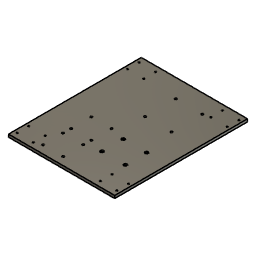
Base roulante (Autodesk Fusion 360 design; units mm, degrees)
Autodesk Fusion 360 part; units mm, degrees
sketch "Sketch1" plane through (0, 0, 0) normal (0, 1, 0) x (1, 0, 0)
  line L0 (0, 0) -> (200, 0)
  line L1 (200, 0) -> (200, 250)
  line L2 (200, 250) -> (0, 250)
  line L3 (0, 250) -> (0, 0)
  circle A0 centre (6, 240) radius 1.5
  circle A1 centre (37, 240) radius 1.5
  line L4 (100, 250) -> (100, 0)
  line L5 (0, 125) -> (200, 125)
  circle A2 centre (163, 240) radius 1.5
  circle A3 centre (194, 240) radius 1.5
  circle A4 centre (6, 10) radius 1.5
  circle A5 centre (163, 10) radius 1.5
  circle A6 centre (37, 10) radius 1.5
  circle A7 centre (194, 10) radius 1.5
  circle A8 centre (6, 218) radius 1.5
  circle A9 centre (37, 218) radius 1.5
  circle A10 centre (163, 218) radius 1.5
  circle A11 centre (194, 218) radius 1.5
  circle A12 centre (37, 32) radius 1.5
  circle A13 centre (6, 32) radius 1.5
  circle A14 centre (194, 32) radius 1.5
  circle A15 centre (163, 32) radius 1.5
  line L6 (34.25, 238.4123) -> (37, 236.8246)
  line L7 (37, 236.8246) -> (39.75, 238.4123)
  line L8 (39.75, 238.4123) -> (39.75, 241.5877)
  line L9 (39.75, 241.5877) -> (37, 243.1754)
  line L10 (37, 243.1754) -> (34.25, 241.5877)
  line L11 (34.25, 241.5877) -> (34.25, 238.4123)
  line L12 (8.75, 238.4123) -> (8.75, 241.5877)
  line L13 (8.75, 241.5877) -> (6, 243.1754)
  line L14 (6, 243.1754) -> (3.25, 241.5877)
  line L15 (3.25, 241.5877) -> (3.25, 238.4123)
  line L16 (3.25, 238.4123) -> (6, 236.8246)
  line L17 (6, 236.8246) -> (8.75, 238.4123)
  line L18 (34.25, 219.5877) -> (34.25, 216.4123)
  line L19 (34.25, 216.4123) -> (37, 214.8246)
  line L20 (37, 214.8246) -> (39.75, 216.4123)
  line L21 (39.75, 216.4123) -> (39.75, 219.5877)
  line L22 (39.75, 219.5877) -> (37, 221.1754)
  line L23 (37, 221.1754) -> (34.25, 219.5877)
  line L24 (3.25, 219.5877) -> (3.25, 216.4123)
  line L25 (3.25, 216.4123) -> (6, 214.8246)
  line L26 (6, 214.8246) -> (8.75, 216.4123)
  line L27 (8.75, 216.4123) -> (8.75, 219.5877)
  line L28 (8.75, 219.5877) -> (6, 221.1754)
  line L29 (6, 221.1754) -> (3.25, 219.5877)
  line L30 (191.25, 238.4123) -> (191.25, 241.5877)
  line L31 (194, 214.8246) -> (191.25, 216.4123)
  line L32 (160.25, 219.5877) -> (163, 221.1754)
  line L33 (163, 214.8246) -> (160.25, 216.4123)
  line L34 (163, 236.8246) -> (160.25, 238.4123)
  line L35 (194, 221.1754) -> (196.75, 219.5877)
  line L36 (191.25, 219.5877) -> (194, 221.1754)
  line L37 (196.75, 219.5877) -> (196.75, 216.4123)
  line L38 (194, 236.8246) -> (191.25, 238.4123)
  line L39 (160.25, 238.4123) -> (160.25, 241.5877)
  line L40 (160.25, 216.4123) -> (160.25, 219.5877)
  line L41 (196.75, 238.4123) -> (194, 236.8246)
  line L42 (196.75, 216.4123) -> (194, 214.8246)
  line L43 (160.25, 241.5877) -> (163, 243.1754)
  line L44 (165.75, 219.5877) -> (165.75, 216.4123)
  line L45 (196.75, 241.5877) -> (196.75, 238.4123)
  line L46 (163, 221.1754) -> (165.75, 219.5877)
  line L47 (165.75, 216.4123) -> (163, 214.8246)
  line L48 (194, 243.1754) -> (196.75, 241.5877)
  line L49 (191.25, 216.4123) -> (191.25, 219.5877)
  line L50 (165.75, 238.4123) -> (163, 236.8246)
  line L51 (191.25, 241.5877) -> (194, 243.1754)
  line L52 (163, 243.1754) -> (165.75, 241.5877)
  line L53 (165.75, 241.5877) -> (165.75, 238.4123)
  line L54 (8.75, 33.5877) -> (8.75, 30.4123)
  line L55 (37, 28.8246) -> (34.25, 30.4123)
  line L56 (34.25, 8.4123) -> (34.25, 11.5877)
  line L57 (37, 35.1754) -> (39.75, 33.5877)
  line L58 (6, 35.1754) -> (8.75, 33.5877)
  line L59 (34.25, 33.5877) -> (37, 35.1754)
  line L60 (37, 6.8246) -> (34.25, 8.4123)
  line L61 (3.25, 8.4123) -> (3.25, 11.5877)
  line L62 (39.75, 11.5877) -> (39.75, 8.4123)
  line L63 (6, 13.1754) -> (8.75, 11.5877)
  line L64 (37, 13.1754) -> (39.75, 11.5877)
  line L65 (39.75, 8.4123) -> (37, 6.8246)
  line L66 (39.75, 30.4123) -> (37, 28.8246)
  line L67 (8.75, 11.5877) -> (8.75, 8.4123)
  line L68 (8.75, 30.4123) -> (6, 28.8246)
  line L69 (34.25, 11.5877) -> (37, 13.1754)
  line L70 (3.25, 30.4123) -> (3.25, 33.5877)
  line L71 (34.25, 30.4123) -> (34.25, 33.5877)
  line L72 (8.75, 8.4123) -> (6, 6.8246)
  line L73 (3.25, 33.5877) -> (6, 35.1754)
  line L74 (6, 6.8246) -> (3.25, 8.4123)
  line L75 (39.75, 33.5877) -> (39.75, 30.4123)
  line L76 (6, 28.8246) -> (3.25, 30.4123)
  line L77 (3.25, 11.5877) -> (6, 13.1754)
  line L78 (191.25, 8.4123) -> (194, 6.8246)
  line L79 (165.75, 11.5877) -> (163, 13.1754)
  line L80 (194, 6.8246) -> (196.75, 8.4123)
  line L81 (165.75, 30.4123) -> (165.75, 33.5877)
  line L82 (163, 28.8246) -> (165.75, 30.4123)
  line L83 (196.75, 11.5877) -> (194, 13.1754)
  line L84 (191.25, 30.4123) -> (194, 28.8246)
  line L85 (194, 13.1754) -> (191.25, 11.5877)
  line L86 (196.75, 33.5877) -> (194, 35.1754)
  line L87 (165.75, 33.5877) -> (163, 35.1754)
  line L88 (194, 35.1754) -> (191.25, 33.5877)
  line L89 (165.75, 8.4123) -> (165.75, 11.5877)
  line L90 (160.25, 11.5877) -> (160.25, 8.4123)
  line L91 (196.75, 30.4123) -> (196.75, 33.5877)
  line L92 (163, 6.8246) -> (165.75, 8.4123)
  line L93 (160.25, 33.5877) -> (160.25, 30.4123)
  line L94 (163, 13.1754) -> (160.25, 11.5877)
  line L95 (191.25, 11.5877) -> (191.25, 8.4123)
  line L96 (196.75, 8.4123) -> (196.75, 11.5877)
  line L97 (160.25, 30.4123) -> (163, 28.8246)
  line L98 (160.25, 8.4123) -> (163, 6.8246)
  line L99 (191.25, 33.5877) -> (191.25, 30.4123)
  line L100 (163, 35.1754) -> (160.25, 33.5877)
  line L101 (194, 28.8246) -> (196.75, 30.4123)
  point P0 (37, 240)
  point P1 (6, 240)
  point P2 (37, 218)
  point P3 (6, 218)
  point P4 (194, 240)
  point P5 (163, 218)
  point P6 (163, 218)
  point P7 (194, 240)
  point P8 (194, 218)
  point P9 (6, 10)
  point P10 (37, 10)
  point P11 (37, 10)
  point P12 (6, 32)
  point P13 (6, 10)
  point P14 (6, 32)
  point P15 (37, 32)
  point P16 (37, 32)
  point P17 (194, 10)
  point P18 (163, 10)
  point P19 (194, 32)
  point P20 (163, 32)
  point P21 (163, 32)
  point P22 (194, 32)
  point P23 (194, 10)
  point P24 (163, 32)
  point P25 (194, 10)
  dimension "d1" = 200
  dimension "d2" = 250
  dimension "d3" = 3
  dimension "d4" = 6
  dimension "d5" = 10
  dimension "d6" = 3
  dimension "d8" = 10
  dimension "d11" = 3
  dimension "d12" = 3
  dimension "d13" = 32
  dimension "d14" = 32
  dimension "d15" = 6
  dimension "d16" = 31
  dimension "d17" = 31
  dimension "d19" = 2.75
  dimension "d20" = 2.75
  dimension "d21" = 2.75
  dimension "d22" = 2.75
  constraint horizontal L0
  constraint vertical L1
  constraint horizontal L2
  constraint vertical L3
  constraint coincident L0.start L3.end
  constraint midpoint L2 L4.start
  constraint midpoint L0 L4.end
  constraint midpoint L3 L5.start
  constraint midpoint L1 L5.end
  constraint symmetric A0 L4 A3
  constraint symmetric A1 L4 A2
  constraint symmetric A0 L5 A4
  constraint symmetric A1 L5 A6
  constraint symmetric L5 A2 A5
  constraint symmetric L5 A3 A7
  constraint symmetric L4 A8 A11
  constraint symmetric L4 A9 A10
  constraint symmetric L5 A8 A13
  constraint symmetric L5 A9 A12
  constraint symmetric L5 A10 A15
  constraint symmetric L5 A11 A14
  constraint coincident P0 A1.centre
  constraint coincident P1 A0.centre
  constraint coincident P2 A9.centre
  constraint coincident P3 A8.centre
  constraint parallel L3 L15
  constraint parallel L11 L12
  constraint parallel L18 L27
  constraint parallel L3 L24
  constraint symmetric P1 L4 P7
  constraint symmetric L4 P2 P6
  constraint symmetric L4 L6.start L50.start
  constraint symmetric L4 L6.end L34.start
  constraint symmetric L4 L7.end L34.end
  constraint symmetric L4 L8.end L39.end
  constraint symmetric L4 L9.end L43.end
  constraint symmetric L4 L10.end L52.end
  constraint symmetric L4 L12.start L30.start
  constraint symmetric L4 L12.end L30.end
  constraint symmetric L4 L13.end L48.start
  constraint symmetric L4 L14.end L45.start
  constraint symmetric L4 L15.end L41.start
  constraint symmetric L4 L16.end L38.start
  constraint symmetric L4 P1 P7
  constraint symmetric L4 L18.start L44.start
  constraint symmetric L4 L18.end L44.end
  constraint symmetric L4 L19.end L33.start
  constraint symmetric L4 L20.end L33.end
  constraint symmetric L4 L21.end L32.start
  constraint symmetric L4 L22.end L32.end
  constraint symmetric L4 L24.start L35.end
  constraint symmetric L4 L24.end L37.end
  constraint symmetric L4 L25.end L31.start
  constraint symmetric L4 L26.end L31.end
  constraint symmetric L4 L27.end L36.start
  constraint symmetric L4 L28.end L35.start
  constraint symmetric L4 P3 P8
  constraint symmetric P1 L5 P13
  constraint symmetric P0 L5 P11
  constraint symmetric L5 P7 P25
  constraint symmetric L5 A2.centre P18
  constraint symmetric L5 P3 P14
  constraint symmetric L5 P2 P16
  constraint symmetric L5 P6 P24
  constraint symmetric L5 P8 P22
  constraint symmetric L5 L6.start L56.end
  constraint symmetric L5 L6.end L64.start
  constraint symmetric L5 L7.end L62.start
  constraint symmetric L5 L8.end L62.end
  constraint symmetric L5 L9.end L60.start
  constraint symmetric L5 L10.end L56.start
  constraint symmetric L5 P0 P11
  constraint symmetric L5 L12.start L63.end
  constraint symmetric L5 L12.end L67.end
  constraint symmetric L5 L13.end L72.end
  constraint symmetric L5 L14.end L61.start
  constraint symmetric L5 L15.end L61.end
  constraint symmetric L5 L16.end L63.start
  constraint symmetric L5 P1 P13
  constraint symmetric L5 L18.start L55.end
  constraint symmetric L5 L18.end L59.start
  constraint symmetric L5 L19.end L57.start
  constraint symmetric L5 L20.end L57.end
  constraint symmetric L5 L21.end L66.start
  constraint symmetric L5 L22.end L55.start
  constraint symmetric L5 L24.start L70.start
  constraint symmetric L5 L24.end L70.end
  constraint symmetric L5 L25.end L58.start
  constraint symmetric L5 L26.end L54.start
  constraint symmetric L5 L27.end L54.end
  constraint symmetric L5 L28.end L68.end
  constraint symmetric L5 L35.start L84.end
  constraint symmetric L5 L36.start L84.start
  constraint symmetric L5 L31.end L88.end
  constraint symmetric L5 L32.end L82.start
  constraint symmetric L5 L32.start L93.end
  constraint symmetric L5 L43.end L92.start
  constraint symmetric L5 L30.start L85.end
  constraint symmetric L5 L34.start L79.end
  constraint symmetric L5 L52.end L89.start
  constraint symmetric L5 L33.start L87.end
  constraint symmetric L5 L38.start L83.end
  constraint symmetric L5 L30.end L78.start
  constraint symmetric L5 L44.start L81.start
  constraint symmetric L5 L33.end L93.start
  constraint symmetric L5 L48.start L78.end
  constraint symmetric L5 L44.end L81.end
  constraint symmetric L5 L34.end L90.start
  constraint symmetric L5 L39.end L90.end
  constraint symmetric L5 L50.start L79.start
  constraint symmetric L5 L31.start L86.end
  constraint symmetric L5 L35.end L91.start
  constraint symmetric L5 L37.end L86.start
  constraint symmetric L5 L41.start L83.start
  constraint symmetric L5 L45.start L80.end
  measures "d1" distance of L0.start L0.end
  measures "d2" distance of L0.start L2.end
  measures "d3" diameter of A0
  measures "d4" distance of L3 P1
  measures "d5" distance of L2 P1
  measures "d6" diameter of A1
  measures "d8" distance of L2 P0
  measures "d11" diameter of A8
  measures "d12" diameter of A9
  measures "d13" distance of L2 P3
  measures "d14" distance of L2 P2
  measures "d15" distance of L3 P3
  measures "d16" distance of P1 P0
  measures "d17" distance of P3 P2
  measures "d19" distance of P0 L11
  measures "d20" distance of P1 L17
  measures "d21" distance of P2 L23
  measures "d22" distance of P3 L29
extrude "Extrude1" add sketch "Sketch1" along normal blind 5 contours L0 L3 L4 L5 | L0 L1 L4 L5 | L2 L3 L4 L5 | L1 L2 L4 L5 | L6 L7 L8 L9 L10 L11 | L12 L13 L14 L15 L16 L17 | L18 L19 L20 L21 L22 L23 | L24 L25 L26 L27 L28 L29 | L30 L38 L41 L45 L48 L51 | L31 L35 L36 L37 L42 L49 | L32 L33 L40 L44 L46 L47 | L34 L39 L43 L50 L52 L53 | L54 L58 L68 L70 L73 L76 | L55 L57 L59 L66 L71 L75 | L56 L60 L62 L64 L65 L69 | L61 L63 L67 L72 L74 L77 | L78 L80 L83 L85 L95 L96 | L79 L89 L90 L92 L94 L98 | L81 L82 L87 L93 L97 L100 | L84 L86 L88 L91 L99 L101
extrude "Extrude2" cut sketch "Sketch1" along normal blind 2.4 contours A12 | A13 | L6 L7 L8 L9 L10 L11 | L12 L13 L14 L15 L16 L17 | L18 L19 L20 L21 L22 L23 | L24 L25 L26 L27 L28 L29 | L30 L38 L41 L45 L48 L51 | L31 L35 L36 L37 L42 L49 | L32 L33 L40 L44 L46 L47 | L34 L39 L43 L50 L52 L53 | L54 L58 L68 L70 L73 L76 | L55 L57 L59 L66 L71 L75 | L56 L60 L62 L64 L65 L69 | L61 L63 L67 L72 L74 L77 | L78 L80 L83 L85 L95 L96 | L79 L89 L90 L92 L94 L98 | L81 L82 L87 L93 L97 L100 | L84 L86 L88 L91 L99 L101
sketch "Sketch2" plane through (0, 0, 0) normal (0, -1, 0) x (1, 0, 0)
  line L0 (6, -13.1754) -> (3.25, -11.5877)
  line L1 (3.25, -11.5877) -> (3.25, -8.4123)
  line L2 (3.25, -8.4123) -> (6, -6.8246)
  line L3 (6, -6.8246) -> (8.75, -8.4123)
  line L4 (8.75, -8.4123) -> (8.75, -11.5877)
  line L5 (8.75, -11.5877) -> (6, -13.1754)
  line L6 (165.75, -33.5877) -> (163, -35.1754)
  line L7 (163, -35.1754) -> (160.25, -33.5877)
  line L8 (160.25, -33.5877) -> (160.25, -30.4123)
  line L9 (160.25, -30.4123) -> (163, -28.8246)
  line L10 (163, -28.8246) -> (165.75, -30.4123)
  line L11 (165.75, -30.4123) -> (165.75, -33.5877)
  line L12 (37, -243.1754) -> (34.25, -241.5877)
  line L13 (34.25, -241.5877) -> (34.25, -238.4123)
  line L14 (34.25, -238.4123) -> (37, -236.8246)
  line L15 (37, -236.8246) -> (39.75, -238.4123)
  line L16 (39.75, -238.4123) -> (39.75, -241.5877)
  line L17 (39.75, -241.5877) -> (37, -243.1754)
  line L18 (191.25, -219.5877) -> (191.25, -216.4123)
  line L19 (191.25, -216.4123) -> (194, -214.8246)
  line L20 (194, -214.8246) -> (196.75, -216.4123)
  line L21 (196.75, -216.4123) -> (196.75, -219.5877)
  line L22 (196.75, -219.5877) -> (194, -221.1754)
  line L23 (194, -221.1754) -> (191.25, -219.5877)
  line L24 (163, -214.8246) -> (165.75, -216.4123)
  line L25 (165.75, -216.4123) -> (165.75, -219.5877)
  line L26 (165.75, -219.5877) -> (163, -221.1754)
  line L27 (163, -221.1754) -> (160.25, -219.5877)
  line L28 (160.25, -219.5877) -> (160.25, -216.4123)
  line L29 (160.25, -216.4123) -> (163, -214.8246)
  line L30 (39.75, -219.5877) -> (37, -221.1754)
  line L31 (37, -221.1754) -> (34.25, -219.5877)
  line L32 (34.25, -219.5877) -> (34.25, -216.4123)
  line L33 (34.25, -216.4123) -> (37, -214.8246)
  line L34 (37, -214.8246) -> (39.75, -216.4123)
  line L35 (39.75, -216.4123) -> (39.75, -219.5877)
  line L36 (194, -6.8246) -> (196.75, -8.4123)
  line L37 (196.75, -8.4123) -> (196.75, -11.5877)
  line L38 (196.75, -11.5877) -> (194, -13.1754)
  line L39 (194, -13.1754) -> (191.25, -11.5877)
  line L40 (191.25, -11.5877) -> (191.25, -8.4123)
  line L41 (191.25, -8.4123) -> (194, -6.8246)
  line L42 (37, -13.1754) -> (34.25, -11.5877)
  line L43 (34.25, -11.5877) -> (34.25, -8.4123)
  line L44 (34.25, -8.4123) -> (37, -6.8246)
  line L45 (37, -6.8246) -> (39.75, -8.4123)
  line L46 (39.75, -8.4123) -> (39.75, -11.5877)
  line L47 (39.75, -11.5877) -> (37, -13.1754)
  line L48 (3.25, -30.4123) -> (6, -28.8246)
  line L49 (6, -28.8246) -> (8.75, -30.4123)
  line L50 (8.75, -30.4123) -> (8.75, -33.5877)
  line L51 (8.75, -33.5877) -> (6, -35.1754)
  line L52 (6, -35.1754) -> (3.25, -33.5877)
  line L53 (3.25, -33.5877) -> (3.25, -30.4123)
  line L54 (191.25, -30.4123) -> (194, -28.8246)
  line L55 (194, -28.8246) -> (196.75, -30.4123)
  line L56 (196.75, -30.4123) -> (196.75, -33.5877)
  line L57 (196.75, -33.5877) -> (194, -35.1754)
  line L58 (194, -35.1754) -> (191.25, -33.5877)
  line L59 (191.25, -33.5877) -> (191.25, -30.4123)
  line L60 (3.25, -238.4123) -> (6, -236.8246)
  line L61 (6, -236.8246) -> (8.75, -238.4123)
  line L62 (8.75, -238.4123) -> (8.75, -241.5877)
  line L63 (8.75, -241.5877) -> (6, -243.1754)
  line L64 (6, -243.1754) -> (3.25, -241.5877)
  line L65 (3.25, -241.5877) -> (3.25, -238.4123)
  line L66 (194, -243.1754) -> (191.25, -241.5877)
  line L67 (191.25, -241.5877) -> (191.25, -238.4123)
  line L68 (191.25, -238.4123) -> (194, -236.8246)
  line L69 (194, -236.8246) -> (196.75, -238.4123)
  line L70 (196.75, -238.4123) -> (196.75, -241.5877)
  line L71 (196.75, -241.5877) -> (194, -243.1754)
  line L72 (165.75, -238.4123) -> (165.75, -241.5877)
  line L73 (165.75, -241.5877) -> (163, -243.1754)
  line L74 (163, -243.1754) -> (160.25, -241.5877)
  line L75 (160.25, -241.5877) -> (160.25, -238.4123)
  line L76 (160.25, -238.4123) -> (163, -236.8246)
  line L77 (163, -236.8246) -> (165.75, -238.4123)
  line L78 (8.75, -219.5877) -> (6, -221.1754)
  line L79 (6, -221.1754) -> (3.25, -219.5877)
  line L80 (3.25, -219.5877) -> (3.25, -216.4123)
  line L81 (3.25, -216.4123) -> (6, -214.8246)
  line L82 (6, -214.8246) -> (8.75, -216.4123)
  line L83 (8.75, -216.4123) -> (8.75, -219.5877)
  line L84 (160.25, -11.5877) -> (160.25, -8.4123)
  line L85 (160.25, -8.4123) -> (163, -6.8246)
  line L86 (163, -6.8246) -> (165.75, -8.4123)
  line L87 (165.75, -8.4123) -> (165.75, -11.5877)
  line L88 (165.75, -11.5877) -> (163, -13.1754)
  line L89 (163, -13.1754) -> (160.25, -11.5877)
  line L90 (39.75, -30.4123) -> (39.75, -33.5877)
  line L91 (39.75, -33.5877) -> (37, -35.1754)
  line L92 (37, -35.1754) -> (34.25, -33.5877)
  line L93 (34.25, -33.5877) -> (34.25, -30.4123)
  line L94 (34.25, -30.4123) -> (37, -28.8246)
  line L95 (37, -28.8246) -> (39.75, -30.4123)
  line L96 (0, 0) -> (0, -250)
  line L97 (0, -250) -> (200, -250)
  line L98 (200, -250) -> (200, 0)
  line L99 (200, 0) -> (0, 0)
  circle A0 centre (160, -60) radius 2
  circle A1 centre (116, -60) radius 2
  circle A2 centre (160, -100) radius 2
  circle A3 centre (116, -100) radius 2
  circle A4 centre (50, -15) radius 2
  circle A5 centre (88, -15) radius 2
  circle A6 centre (87.486, -53) radius 2
  circle A7 centre (49.486, -52.9965) radius 2
  circle A8 centre (50, -67.9965) radius 2
  circle A9 centre (88, -68) radius 2
  circle A10 centre (88, -106) radius 2
  circle A11 centre (50, -105.9965) radius 2
  circle A12 centre (150, -215) radius 2
  circle A13 centre (100, -215) radius 2
  circle A14 centre (150, -157) radius 2
  circle A15 centre (100, -157) radius 2
  line L100 (118.75, -61.5877) -> (118.75, -58.4123)
  line L101 (118.75, -58.4123) -> (116, -56.8246)
  line L102 (116, -56.8246) -> (113.25, -58.4123)
  line L103 (113.25, -58.4123) -> (113.25, -61.5877)
  line L104 (113.25, -61.5877) -> (116, -63.1754)
  line L105 (116, -63.1754) -> (118.75, -61.5877)
  line L106 (162.75, -61.5877) -> (162.75, -58.4123)
  line L107 (162.75, -58.4123) -> (160, -56.8246)
  line L108 (160, -56.8246) -> (157.25, -58.4123)
  line L109 (157.25, -58.4123) -> (157.25, -61.5877)
  line L110 (157.25, -61.5877) -> (160, -63.1754)
  line L111 (160, -63.1754) -> (162.75, -61.5877)
  line L112 (118.75, -101.5877) -> (118.75, -98.4123)
  line L113 (118.75, -98.4123) -> (116, -96.8246)
  line L114 (116, -96.8246) -> (113.25, -98.4123)
  line L115 (113.25, -98.4123) -> (113.25, -101.5877)
  line L116 (113.25, -101.5877) -> (116, -103.1754)
  line L117 (116, -103.1754) -> (118.75, -101.5877)
  line L118 (160, -103.1754) -> (162.75, -101.5877)
  line L119 (162.75, -101.5877) -> (162.75, -98.4123)
  line L120 (162.75, -98.4123) -> (160, -96.8246)
  line L121 (160, -96.8246) -> (157.25, -98.4123)
  line L122 (157.25, -98.4123) -> (157.25, -101.5877)
  line L123 (157.25, -101.5877) -> (160, -103.1754)
  point P0 (116, -60)
  point P1 (160, -60)
  point P2 (116, -100)
  point P3 (160, -100)
  dimension "d25" = 4
  dimension "d26" = 60
  dimension "d27" = 4
  dimension "d28" = 60
  dimension "d29" = 44
  dimension "d30" = 40
  dimension "d31" = 4
  dimension "d32" = 4
  dimension "d33" = 40
  dimension "d34" = 40
  dimension "d35" = 44
  dimension "d36" = 40
  dimension "d37" = 4
  dimension "d38" = 4
  dimension "d39" = 15
  dimension "d40" = 15
  dimension "d41" = 50
  dimension "d42" = 38
  dimension "d43" = 4
  dimension "d44" = 4
  dimension "d45" = 38
  dimension "d46" = 38
  dimension "d47" = 38
  dimension "d48" = 4
  dimension "d49" = 4
  dimension "d50" = 4
  dimension "d51" = 4
  dimension "d52" = 38
  dimension "d53" = 38
  dimension "d54" = 50
  dimension "d55" = 50
  dimension "d56" = 38
  dimension "d57" = 38
  dimension "d58" = 15
  dimension "d60" = 15
  dimension "d61" = 4
  dimension "d62" = 4
  dimension "d63" = 4
  dimension "d64" = 4
  dimension "d65" = 50
  dimension "d66" = 50
  dimension "d67" = 58
  dimension "d68" = 58
  dimension "d69" = 50
  dimension "d70" = 50
  dimension "d71" = 35
  dimension "d74" = 2.75
  dimension "d75" = 2.75
  dimension "d76" = 2.75
  dimension "d77" = 2.75
  constraint coincident P0 A1.centre
  constraint coincident P1 A0.centre
  constraint coincident P2 A3.centre
  constraint coincident P3 A2.centre
  constraint parallel L98 L106
  constraint parallel L98 L119
  constraint parallel L100 L109
  constraint parallel L112 L122
  measures "d25" diameter of A0
  measures "d26" distance of L99 P1
  measures "d27" diameter of A1
  measures "d28" distance of L99 P0
  measures "d29" distance of P1 P0
  measures "d30" distance of L98 P1
  measures "d31" diameter of A2
  measures "d32" diameter of A3
  measures "d33" vertical distance of P1 P3
  measures "d34" vertical distance of P0 P2
  measures "d35" distance of P3 P2
  measures "d36" distance of L98 P3
  measures "d37" diameter of A4
  measures "d38" diameter of A5
  measures "d39" distance of L99 A5.centre
  measures "d40" distance of L99 A4.centre
  measures "d41" distance of L96 A4.centre
  measures "d42" distance of A4.centre A5.centre
  measures "d43" diameter of A6
  measures "d44" diameter of A7
  measures "d45" vertical distance of A5.centre A6.centre
  measures "d46" horizontal distance of A6.centre A7.centre
  measures "d47" distance of A4.centre A7.centre
  measures "d48" diameter of A8
  measures "d49" diameter of A9
  measures "d50" diameter of A10
  measures "d51" diameter of A11
  measures "d52" horizontal distance of A8.centre A9.centre
  measures "d53" horizontal distance of A10.centre A11.centre
  measures "d54" distance of L96 A8.centre
  measures "d55" distance of L96 A11.centre
  measures "d56" distance of A8.centre A11.centre
  measures "d57" distance of A9.centre A10.centre
  measures "d58" vertical distance of A7.centre A8.centre
  measures "d60" vertical distance of A6.centre A9.centre
  measures "d61" diameter of A12
  measures "d62" diameter of A13
  measures "d63" diameter of A14
  measures "d64" diameter of A15
  measures "d65" horizontal distance of A12.centre A13.centre
  measures "d66" distance of A14.centre A15.centre
  measures "d67" vertical distance of A12.centre A14.centre
  measures "d68" vertical distance of A13.centre A15.centre
  measures "d69" distance of L98 A12.centre
  measures "d70" distance of L98 A14.centre
  measures "d71" distance of L97 A12.centre
  measures "d74" distance of P0 L105
  measures "d75" distance of P1 L111
  measures "d76" distance of P2 L117
  measures "d77" distance of P3 L123
extrude "Extrude3" cut sketch "Sketch2" against normal blind 40 contours A0 | A1 | A2 | A3 | A4 | A5 | A6 | A7 | A8 | A9 | A10 | A11 | A12 | A13 | A14 | A15
extrude "Extrude4" cut sketch "Sketch2" along normal blind 2.4 from surface at -5 contours L100 L101 L102 L103 L104 L105 | L106 L107 L108 L109 L110 L111 | L112 L113 L114 L115 L116 L117 | L118 L119 L120 L121 L122 L123
